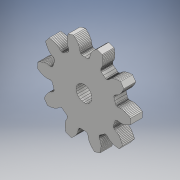
# Autodesk Inventor part: Engranajes PEQUENO final 2017
Saved by Autodesk Inventor 2017 (Build 210142000, 142)
## iProperties
Created: 2017-09-24
Part Number: Engranajes PEQUENO final 2017
Material: Generic
Document SubType Name: Modeling
Designer: ANDRES
Density: 1 g/cm^3
Appearance: Default
Author: ANDRES
## iProperties of the stored document Engranajes PEQUENO final 2017_3DPrint.ipt
Created: 2017-09-24
Part Number: Engranajes PEQUENO final 2017_3DPrint
Material: Generic
Document SubType Name: Modeling
Designer: ANDRES
Density: 1 g/cm^3
Appearance: Default
Author: ANDRES
Autodesk Inventor part; units mm, degrees
ref_plane "YZ Plane" through (0, 0, 0) normal (1, 0, 0) x (0, 1, 0)
ref_plane "XZ Plane" through (0, 0, 0) normal (0, 1, 0) x (-1, 0, 0)
ref_plane "XY Plane" through (0, 0, 0) normal (0, 0, 1) x (1, 0, 0)
sketch "Sketch1" plane through (0, 0, 0) normal (0, 1, 0) x (-1, 0, 0)
  line L0 (3.2222, 8) -> (3.1344, 8.1445)
  line L1 (3.1344, 8.1445) -> (3.0716, 8.1935)
  line L2 (3.0716, 8.1935) -> (3.0129, 8.2255)
  line L3 (3.0129, 8.2255) -> (2.9568, 8.2486)
  line L4 (2.9568, 8.2486) -> (2.902, 8.2657)
  line L5 (2.902, 8.2657) -> (2.8484, 8.2779)
  line L6 (2.8484, 8.2779) -> (2.7432, 8.2923)
  line L7 (2.7432, 8.2923) -> (2.6406, 8.2961)
  line L8 (2.6406, 8.2961) -> (2.5395, 8.2918)
  line L9 (2.5395, 8.2918) -> (2.3414, 8.2639)
  line L10 (2.3414, 8.2639) -> (2.1473, 8.2146)
  line L11 (2.1473, 8.2146) -> (1.9461, 8.2027)
  line L12 (1.9461, 8.2027) -> (1.7394, 8.2197)
  line L13 (1.7394, 8.2197) -> (1.5296, 8.2547)
  line L14 (1.5296, 8.2547) -> (1.318, 8.3058)
  line L15 (1.318, 8.3058) -> (1.1049, 8.3713)
  line L16 (1.1049, 8.3713) -> (0.8908, 8.4503)
  line L17 (0.8908, 8.4503) -> (0.6767, 8.5423)
  line L18 (0.6767, 8.5423) -> (0.4623, 8.6469)
  line L19 (0.4623, 8.6469) -> (0.2484, 8.7638)
  line L20 (0.2484, 8.7638) -> (0.0358, 8.8928)
  line L21 (0.0358, 8.8928) -> (0.0061, 10.0714)
  line L22 (0.0061, 10.0714) -> (0.2121, 10.2108)
  line L23 (0.2121, 10.2108) -> (0.4199, 10.3383)
  line L24 (0.4199, 10.3383) -> (0.6284, 10.4534)
  line L25 (0.6284, 10.4534) -> (0.8379, 10.5562)
  line L26 (0.8379, 10.5562) -> (1.0478, 10.6459)
  line L27 (1.0478, 10.6459) -> (1.2573, 10.7218)
  line L28 (1.2573, 10.7218) -> (1.4661, 10.7836)
  line L29 (1.4661, 10.7836) -> (1.6739, 10.8293)
  line L30 (1.6739, 10.8293) -> (1.8793, 10.8565)
  line L31 (1.8793, 10.8565) -> (2.081, 10.8547)
  line L32 (2.081, 10.8547) -> (2.2771, 10.8153)
  line L33 (2.2771, 10.8153) -> (2.4765, 10.7973)
  line L34 (2.4765, 10.7973) -> (2.5776, 10.798)
  line L35 (2.5776, 10.798) -> (2.68, 10.8069)
  line L36 (2.68, 10.8069) -> (2.7843, 10.8268)
  line L37 (2.7843, 10.8268) -> (2.8372, 10.8417)
  line L38 (2.8372, 10.8417) -> (2.891, 10.8613)
  line L39 (2.891, 10.8613) -> (2.9461, 10.8872)
  line L40 (2.9461, 10.8872) -> (3.003, 10.9223)
  line L41 (3.003, 10.9223) -> (3.0632, 10.9743)
  line L42 (3.0632, 10.9743) -> (3.1438, 11.1229)
  line L43 (3.1438, 11.1229) -> (3.2763, 11.6439)
  line L44 (3.2763, 11.6439) -> (3.4498, 12.1524)
  line L45 (3.4498, 12.1524) -> (3.4635, 12.321)
  line L46 (3.4635, 12.321) -> (3.4417, 12.3975)
  line L47 (3.4417, 12.3975) -> (3.4133, 12.4579)
  line L48 (3.4133, 12.4579) -> (3.3812, 12.5098)
  line L49 (3.3812, 12.5098) -> (3.347, 12.5555)
  line L50 (3.347, 12.5555) -> (3.3106, 12.5971)
  line L51 (3.3106, 12.5971) -> (3.2342, 12.6705)
  line L52 (3.2342, 12.6705) -> (3.1534, 12.734)
  line L53 (3.1534, 12.734) -> (3.0691, 12.7899)
  line L54 (3.0691, 12.7899) -> (2.8923, 12.8836)
  line L55 (2.8923, 12.8836) -> (2.7064, 12.9578)
  line L56 (2.7064, 12.9578) -> (2.5364, 13.0665)
  line L57 (2.5364, 13.0665) -> (2.3792, 13.2017)
  line L58 (2.3792, 13.2017) -> (2.2304, 13.3535)
  line L59 (2.2304, 13.3535) -> (2.0892, 13.5191)
  line L60 (2.0892, 13.5191) -> (1.955, 13.6975)
  line L61 (1.955, 13.6975) -> (1.8283, 13.8872)
  line L62 (1.8283, 13.8872) -> (1.7092, 14.0876)
  line L63 (1.7092, 14.0876) -> (1.5972, 14.2982)
  line L64 (1.5972, 14.2982) -> (1.493, 14.5184)
  line L65 (1.493, 14.5184) -> (1.3967, 14.7477)
  line L66 (1.3967, 14.7477) -> (2.0655, 15.7185)
  line L67 (2.0655, 15.7185) -> (2.3142, 15.7104)
  line L68 (2.3142, 15.7104) -> (2.557, 15.6914)
  line L69 (2.557, 15.6914) -> (2.7935, 15.6619)
  line L70 (2.7935, 15.6619) -> (3.0234, 15.622)
  line L71 (3.0234, 15.622) -> (3.2459, 15.5712)
  line L72 (3.2459, 15.5712) -> (3.46, 15.5095)
  line L73 (3.46, 15.5095) -> (3.6652, 15.4366)
  line L74 (3.6652, 15.4366) -> (3.86, 15.3515)
  line L75 (3.86, 15.3515) -> (4.0424, 15.2527)
  line L76 (4.0424, 15.2527) -> (4.2044, 15.1328)
  line L77 (4.2044, 15.1328) -> (4.3401, 14.9855)
  line L78 (4.3401, 14.9855) -> (4.4907, 14.8539)
  line L79 (4.4907, 14.8539) -> (4.573, 14.7949)
  line L80 (4.573, 14.7949) -> (4.6611, 14.7421)
  line L81 (4.6611, 14.7421) -> (4.7569, 14.6966)
  line L82 (4.7569, 14.6966) -> (4.8087, 14.6776)
  line L83 (4.8087, 14.6776) -> (4.8638, 14.6618)
  line L84 (4.8638, 14.6618) -> (4.9235, 14.6504)
  line L85 (4.9235, 14.6504) -> (4.99, 14.6456)
  line L86 (4.99, 14.6456) -> (5.0695, 14.6522)
  line L87 (5.0695, 14.6522) -> (5.2219, 14.725)
  line L88 (5.2219, 14.725) -> (5.6355, 15.0684)
  line L89 (5.6355, 15.0684) -> (6.0747, 15.3778)
  line L90 (6.0747, 15.3778) -> (6.1849, 15.506)
  line L91 (6.1849, 15.506) -> (6.2121, 15.581)
  line L92 (6.2121, 15.581) -> (6.2245, 15.6467)
  line L93 (6.2245, 15.6467) -> (6.2291, 15.7072)
  line L94 (6.2291, 15.7072) -> (6.2283, 15.7646)
  line L95 (6.2283, 15.7646) -> (6.2234, 15.8195)
  line L96 (6.2234, 15.8195) -> (6.2046, 15.9239)
  line L97 (6.2046, 15.9239) -> (6.1767, 16.0227)
  line L98 (6.1767, 16.0227) -> (6.1411, 16.1174)
  line L99 (6.1411, 16.1174) -> (6.0532, 16.2972)
  line L100 (6.0532, 16.2972) -> (5.9464, 16.4663)
  line L101 (5.9464, 16.4663) -> (5.873, 16.6543)
  line L102 (5.873, 16.6543) -> (5.8249, 16.856)
  line L103 (5.8249, 16.856) -> (5.7937, 17.0663)
  line L104 (5.7937, 17.0663) -> (5.7768, 17.2834)
  line L105 (5.7768, 17.2834) -> (5.773, 17.5064)
  line L106 (5.773, 17.5064) -> (5.7821, 17.7343)
  line L107 (5.7821, 17.7343) -> (5.8034, 17.9664)
  line L108 (5.8034, 17.9664) -> (5.8366, 18.2027)
  line L109 (5.8366, 18.2027) -> (5.8815, 18.4419)
  line L110 (5.8815, 18.4419) -> (5.9383, 18.6843)
  line L111 (5.9383, 18.6843) -> (7.05, 19.0769)
  line L112 (7.05, 19.0769) -> (7.2464, 18.9241)
  line L113 (7.2464, 18.9241) -> (7.4318, 18.7661)
  line L114 (7.4318, 18.7661) -> (7.6059, 18.6031)
  line L115 (7.6059, 18.6031) -> (7.7685, 18.4358)
  line L116 (7.7685, 18.4358) -> (7.9184, 18.2641)
  line L117 (7.9184, 18.2641) -> (8.0556, 18.0883)
  line L118 (8.0556, 18.0883) -> (8.1788, 17.9088)
  line L119 (8.1788, 17.9088) -> (8.2865, 17.7254)
  line L120 (8.2865, 17.7254) -> (8.376, 17.5383)
  line L121 (8.376, 17.5383) -> (8.4367, 17.346)
  line L122 (8.4367, 17.346) -> (8.4599, 17.1471)
  line L123 (8.4599, 17.1471) -> (8.5044, 16.952)
  line L124 (8.5044, 16.952) -> (8.5364, 16.856)
  line L125 (8.5364, 16.856) -> (8.5765, 16.7616)
  line L126 (8.5765, 16.7616) -> (8.6274, 16.6686)
  line L127 (8.6274, 16.6686) -> (8.6581, 16.6226)
  line L128 (8.6581, 16.6226) -> (8.6934, 16.5777)
  line L129 (8.6934, 16.5777) -> (8.7351, 16.5333)
  line L130 (8.7351, 16.5333) -> (8.7859, 16.4901)
  line L131 (8.7859, 16.4901) -> (8.8542, 16.4489)
  line L132 (8.8542, 16.4489) -> (9.0204, 16.4183)
  line L133 (9.0204, 16.4183) -> (9.5568, 16.4532)
  line L134 (9.5568, 16.4532) -> (10.094, 16.4454)
  line L135 (10.094, 16.4454) -> (10.2586, 16.4845)
  line L136 (10.2586, 16.4845) -> (10.3246, 16.529)
  line L137 (10.3246, 16.529) -> (10.3734, 16.5747)
  line L138 (10.3734, 16.5747) -> (10.4125, 16.6212)
  line L139 (10.4125, 16.6212) -> (10.4455, 16.6679)
  line L140 (10.4455, 16.6679) -> (10.474, 16.7152)
  line L141 (10.474, 16.7152) -> (10.5199, 16.8107)
  line L142 (10.5199, 16.8107) -> (10.5555, 16.9072)
  line L143 (10.5555, 16.9072) -> (10.5826, 17.0048)
  line L144 (10.5826, 17.0048) -> (10.6171, 17.2019)
  line L145 (10.6171, 17.2019) -> (10.6301, 17.4015)
  line L146 (10.6301, 17.4015) -> (10.6811, 17.5966)
  line L147 (10.6811, 17.5966) -> (10.7611, 17.7881)
  line L148 (10.7611, 17.7881) -> (10.8593, 17.9766)
  line L149 (10.8593, 17.9766) -> (10.9731, 18.1621)
  line L150 (10.9731, 18.1621) -> (11.1011, 18.3447)
  line L151 (11.1011, 18.3447) -> (11.2425, 18.5238)
  line L152 (11.2425, 18.5238) -> (11.3962, 18.6993)
  line L153 (11.3962, 18.6993) -> (11.5617, 18.8708)
  line L154 (11.5617, 18.8708) -> (11.7391, 19.0379)
  line L155 (11.7391, 19.0379) -> (11.9273, 19.2002)
  line L156 (11.9273, 19.2002) -> (13.0576, 18.8643)
  line L157 (13.0576, 18.8643) -> (13.1264, 18.6251)
  line L158 (13.1264, 18.6251) -> (13.1835, 18.3883)
  line L159 (13.1835, 18.3883) -> (13.2284, 18.1542)
  line L160 (13.2284, 18.1542) -> (13.2614, 17.9233)
  line L161 (13.2614, 17.9233) -> (13.2821, 17.6962)
  line L162 (13.2821, 17.6962) -> (13.2895, 17.4732)
  line L163 (13.2895, 17.4732) -> (13.2837, 17.2555)
  line L164 (13.2837, 17.2555) -> (13.2629, 17.0439)
  line L165 (13.2629, 17.0439) -> (13.2253, 16.8402)
  line L166 (13.2253, 16.8402) -> (13.1613, 16.6487)
  line L167 (13.1613, 16.6487) -> (13.0633, 16.4744)
  line L168 (13.0633, 16.4744) -> (12.9846, 16.2905)
  line L169 (12.9846, 16.2905) -> (12.9541, 16.194)
  line L170 (12.9541, 16.194) -> (12.931, 16.0939)
  line L171 (12.931, 16.0939) -> (12.9176, 15.9887)
  line L172 (12.9176, 15.9887) -> (12.9156, 15.9336)
  line L173 (12.9156, 15.9336) -> (12.9176, 15.8762)
  line L174 (12.9176, 15.8762) -> (12.9252, 15.816)
  line L175 (12.9252, 15.816) -> (12.941, 15.751)
  line L176 (12.941, 15.751) -> (12.972, 15.6776)
  line L177 (12.972, 15.6776) -> (13.0884, 15.5549)
  line L178 (13.0884, 15.5549) -> (13.5428, 15.2682)
  line L179 (13.5428, 15.2682) -> (13.9729, 14.946)
  line L180 (13.9729, 14.946) -> (14.1288, 14.881)
  line L181 (14.1288, 14.881) -> (14.2086, 14.8782)
  line L182 (14.2086, 14.8782) -> (14.2749, 14.8866)
  line L183 (14.2749, 14.8866) -> (14.3341, 14.9011)
  line L184 (14.3341, 14.9011) -> (14.3882, 14.9194)
  line L185 (14.3882, 14.9194) -> (14.439, 14.941)
  line L186 (14.439, 14.941) -> (14.5322, 14.9913)
  line L187 (14.5322, 14.9913) -> (14.6178, 15.0485)
  line L188 (14.6178, 15.0485) -> (14.6968, 15.1115)
  line L189 (14.6968, 15.1115) -> (14.8407, 15.2507)
  line L190 (14.8407, 15.2507) -> (14.9687, 15.4044)
  line L191 (14.9687, 15.4044) -> (15.1244, 15.5324)
  line L192 (15.1244, 15.5324) -> (15.3017, 15.6401)
  line L193 (15.3017, 15.6401) -> (15.4919, 15.7349)
  line L194 (15.4919, 15.7349) -> (15.6931, 15.8182)
  line L195 (15.6931, 15.8182) -> (15.9042, 15.8907)
  line L196 (15.9042, 15.8907) -> (16.1236, 15.9524)
  line L197 (16.1236, 15.9524) -> (16.3512, 16.004)
  line L198 (16.3512, 16.004) -> (16.5859, 16.0455)
  line L199 (16.5859, 16.0455) -> (16.8277, 16.0765)
  line L200 (16.8277, 16.0765) -> (17.0756, 16.0974)
  line L201 (17.0756, 16.0974) -> (17.7923, 15.1612)
  line L202 (17.7923, 15.1612) -> (17.7077, 14.9273)
  line L203 (17.7077, 14.9273) -> (17.6148, 14.7022)
  line L204 (17.6148, 14.7022) -> (17.5135, 14.4863)
  line L205 (17.5135, 14.4863) -> (17.4045, 14.28)
  line L206 (17.4045, 14.28) -> (17.2875, 14.0842)
  line L207 (17.2875, 14.0842) -> (17.1628, 13.8995)
  line L208 (17.1628, 13.8995) -> (17.03, 13.727)
  line L209 (17.03, 13.727) -> (16.889, 13.5677)
  line L210 (16.889, 13.5677) -> (16.7387, 13.425)
  line L211 (16.7387, 13.425) -> (16.5744, 13.3078)
  line L212 (16.5744, 13.3078) -> (16.3925, 13.2242)
  line L213 (16.3925, 13.2242) -> (16.2208, 13.1219)
  line L214 (16.2208, 13.1219) -> (16.1393, 13.0616)
  line L215 (16.1393, 13.0616) -> (16.0619, 12.9941)
  line L216 (16.0619, 12.9941) -> (15.9892, 12.9171)
  line L217 (15.9892, 12.9171) -> (15.9552, 12.8737)
  line L218 (15.9552, 12.8737) -> (15.9232, 12.8261)
  line L219 (15.9232, 12.8261) -> (15.8937, 12.7728)
  line L220 (15.8937, 12.7728) -> (15.8684, 12.7111)
  line L221 (15.8684, 12.7111) -> (15.8503, 12.6336)
  line L222 (15.8503, 12.6336) -> (15.8725, 12.466)
  line L223 (15.8725, 12.466) -> (16.0714, 11.9666)
  line L224 (16.0714, 11.9666) -> (16.2299, 11.4533)
  line L225 (16.2299, 11.4533) -> (16.3181, 11.3088)
  line L226 (16.3181, 11.3088) -> (16.3808, 11.2598)
  line L227 (16.3808, 11.2598) -> (16.4395, 11.2275)
  line L228 (16.4395, 11.2275) -> (16.4956, 11.2046)
  line L229 (16.4956, 11.2046) -> (16.5505, 11.1876)
  line L230 (16.5505, 11.1876) -> (16.6041, 11.1752)
  line L231 (16.6041, 11.1752) -> (16.709, 11.161)
  line L232 (16.709, 11.161) -> (16.8118, 11.1571)
  line L233 (16.8118, 11.1571) -> (16.9129, 11.1615)
  line L234 (16.9129, 11.1615) -> (17.1111, 11.1894)
  line L235 (17.1111, 11.1894) -> (17.3049, 11.2387)
  line L236 (17.3049, 11.2387) -> (17.5063, 11.2504)
  line L237 (17.5063, 11.2504) -> (17.713, 11.2336)
  line L238 (17.713, 11.2336) -> (17.9226, 11.1983)
  line L239 (17.9226, 11.1983) -> (18.1344, 11.1472)
  line L240 (18.1344, 11.1472) -> (18.3475, 11.082)
  line L241 (18.3475, 11.082) -> (18.5614, 11.003)
  line L242 (18.5614, 11.003) -> (18.7758, 10.9108)
  line L243 (18.7758, 10.9108) -> (18.9902, 10.8064)
  line L244 (18.9902, 10.8064) -> (19.2038, 10.6893)
  line L245 (19.2038, 10.6893) -> (19.4166, 10.5605)
  line L246 (19.4166, 10.5605) -> (19.4463, 9.3819)
  line L247 (19.4463, 9.3819) -> (19.2401, 9.243)
  line L248 (19.2401, 9.243) -> (19.0326, 9.1155)
  line L249 (19.0326, 9.1155) -> (18.8238, 9.0001)
  line L250 (18.8238, 9.0001) -> (18.6145, 8.8975)
  line L251 (18.6145, 8.8975) -> (18.4047, 8.8079)
  line L252 (18.4047, 8.8079) -> (18.1951, 8.7319)
  line L253 (18.1951, 8.7319) -> (17.9864, 8.6702)
  line L254 (17.9864, 8.6702) -> (17.7786, 8.6245)
  line L255 (17.7786, 8.6245) -> (17.5731, 8.5973)
  line L256 (17.5731, 8.5973) -> (17.3714, 8.5991)
  line L257 (17.3714, 8.5991) -> (17.1751, 8.6384)
  line L258 (17.1751, 8.6384) -> (16.9759, 8.6565)
  line L259 (16.9759, 8.6565) -> (16.8749, 8.6557)
  line L260 (16.8749, 8.6557) -> (16.7722, 8.6466)
  line L261 (16.7722, 8.6466) -> (16.6681, 8.627)
  line L262 (16.6681, 8.627) -> (16.6153, 8.612)
  line L263 (16.6153, 8.612) -> (16.5614, 8.5925)
  line L264 (16.5614, 8.5925) -> (16.5063, 8.5666)
  line L265 (16.5063, 8.5666) -> (16.4494, 8.5315)
  line L266 (16.4494, 8.5315) -> (16.3892, 8.4792)
  line L267 (16.3892, 8.4792) -> (16.3084, 8.3306)
  line L268 (16.3084, 8.3306) -> (16.1761, 7.8099)
  line L269 (16.1761, 7.8099) -> (16.0024, 7.3014)
  line L270 (16.0024, 7.3014) -> (15.9886, 7.1327)
  line L271 (15.9886, 7.1327) -> (16.0107, 7.0563)
  line L272 (16.0107, 7.0563) -> (16.0392, 6.9958)
  line L273 (16.0392, 6.9958) -> (16.0712, 6.944)
  line L274 (16.0712, 6.944) -> (16.1055, 6.898)
  line L275 (16.1055, 6.898) -> (16.1418, 6.8566)
  line L276 (16.1418, 6.8566) -> (16.2183, 6.7832)
  line L277 (16.2183, 6.7832) -> (16.299, 6.7197)
  line L278 (16.299, 6.7197) -> (16.3834, 6.6638)
  line L279 (16.3834, 6.6638) -> (16.5601, 6.5701)
  line L280 (16.5601, 6.5701) -> (16.7461, 6.4957)
  line L281 (16.7461, 6.4957) -> (16.9157, 6.387)
  line L282 (16.9157, 6.387) -> (17.0732, 6.2519)
  line L283 (17.0732, 6.2519) -> (17.2221, 6.1002)
  line L284 (17.2221, 6.1002) -> (17.3633, 5.9346)
  line L285 (17.3633, 5.9346) -> (17.4974, 5.7563)
  line L286 (17.4974, 5.7563) -> (17.6239, 5.5666)
  line L287 (17.6239, 5.5666) -> (17.7433, 5.3662)
  line L288 (17.7433, 5.3662) -> (17.855, 5.1556)
  line L289 (17.855, 5.1556) -> (17.9594, 4.9354)
  line L290 (17.9594, 4.9354) -> (18.0557, 4.706)
  line L291 (18.0557, 4.706) -> (17.3869, 3.735)
  line L292 (17.3869, 3.735) -> (17.1383, 3.7434)
  line L293 (17.1383, 3.7434) -> (16.8954, 3.7624)
  line L294 (16.8954, 3.7624) -> (16.6587, 3.7919)
  line L295 (16.6587, 3.7919) -> (16.4291, 3.8317)
  line L296 (16.4291, 3.8317) -> (16.2066, 3.8825)
  line L297 (16.2066, 3.8825) -> (15.9925, 3.9443)
  line L298 (15.9925, 3.9443) -> (15.7872, 4.0172)
  line L299 (15.7872, 4.0172) -> (15.5924, 4.1023)
  line L300 (15.5924, 4.1023) -> (15.41, 4.2011)
  line L301 (15.41, 4.2011) -> (15.248, 4.321)
  line L302 (15.248, 4.321) -> (15.1124, 4.4681)
  line L303 (15.1124, 4.4681) -> (14.9618, 4.5999)
  line L304 (14.9618, 4.5999) -> (14.8795, 4.6588)
  line L305 (14.8795, 4.6588) -> (14.7913, 4.7117)
  line L306 (14.7913, 4.7117) -> (14.6956, 4.7571)
  line L307 (14.6956, 4.7571) -> (14.6438, 4.7759)
  line L308 (14.6438, 4.7759) -> (14.5886, 4.7917)
  line L309 (14.5886, 4.7917) -> (14.529, 4.8031)
  line L310 (14.529, 4.8031) -> (14.4624, 4.8082)
  line L311 (14.4624, 4.8082) -> (14.3829, 4.8016)
  line L312 (14.3829, 4.8016) -> (14.2303, 4.7287)
  line L313 (14.2303, 4.7287) -> (13.8171, 4.3852)
  line L314 (13.8171, 4.3852) -> (13.3777, 4.0754)
  line L315 (13.3777, 4.0754) -> (13.2678, 3.9471)
  line L316 (13.2678, 3.9471) -> (13.2406, 3.8722)
  line L317 (13.2406, 3.8722) -> (13.2279, 3.8067)
  line L318 (13.2279, 3.8067) -> (13.2234, 3.746)
  line L319 (13.2234, 3.746) -> (13.2244, 3.6888)
  line L320 (13.2244, 3.6888) -> (13.2292, 3.6339)
  line L321 (13.2292, 3.6339) -> (13.2481, 3.5296)
  line L322 (13.2481, 3.5296) -> (13.276, 3.4308)
  line L323 (13.276, 3.4308) -> (13.3113, 3.3358)
  line L324 (13.3113, 3.3358) -> (13.3995, 3.1562)
  line L325 (13.3995, 3.1562) -> (13.5062, 2.9868)
  line L326 (13.5062, 2.9868) -> (13.5796, 2.7991)
  line L327 (13.5796, 2.7991) -> (13.6274, 2.5972)
  line L328 (13.6274, 2.5972) -> (13.6587, 2.3871)
  line L329 (13.6587, 2.3871) -> (13.6757, 2.1699)
  line L330 (13.6757, 2.1699) -> (13.6793, 1.9469)
  line L331 (13.6793, 1.9469) -> (13.6704, 1.7191)
  line L332 (13.6704, 1.7191) -> (13.6491, 1.4867)
  line L333 (13.6491, 1.4867) -> (13.6159, 1.2507)
  line L334 (13.6159, 1.2507) -> (13.5707, 1.0112)
  line L335 (13.5707, 1.0112) -> (13.5142, 0.7691)
  line L336 (13.5142, 0.7691) -> (12.4025, 0.3764)
  line L337 (12.4025, 0.3764) -> (12.2061, 0.5293)
  line L338 (12.2061, 0.5293) -> (12.0207, 0.6872)
  line L339 (12.0207, 0.6872) -> (11.8464, 0.85)
  line L340 (11.8464, 0.85) -> (11.684, 1.0176)
  line L341 (11.684, 1.0176) -> (11.5339, 1.1893)
  line L342 (11.5339, 1.1893) -> (11.3969, 1.365)
  line L343 (11.3969, 1.365) -> (11.2737, 1.5446)
  line L344 (11.2737, 1.5446) -> (11.166, 1.728)
  line L345 (11.166, 1.728) -> (11.0765, 1.9151)
  line L346 (11.0765, 1.9151) -> (11.0158, 2.1074)
  line L347 (11.0158, 2.1074) -> (10.9926, 2.306)
  line L348 (10.9926, 2.306) -> (10.9481, 2.5013)
  line L349 (10.9481, 2.5013) -> (10.9161, 2.5971)
  line L350 (10.9161, 2.5971) -> (10.876, 2.6918)
  line L351 (10.876, 2.6918) -> (10.8251, 2.7848)
  line L352 (10.8251, 2.7848) -> (10.7944, 2.8305)
  line L353 (10.7944, 2.8305) -> (10.7591, 2.8757)
  line L354 (10.7591, 2.8757) -> (10.7174, 2.9199)
  line L355 (10.7174, 2.9199) -> (10.6664, 2.9633)
  line L356 (10.6664, 2.9633) -> (10.5983, 3.0045)
  line L357 (10.5983, 3.0045) -> (10.4319, 3.0352)
  line L358 (10.4319, 3.0352) -> (9.8957, 3.0002)
  line L359 (9.8957, 3.0002) -> (9.3585, 3.0083)
  line L360 (9.3585, 3.0083) -> (9.1939, 2.9692)
  line L361 (9.1939, 2.9692) -> (9.1279, 2.9245)
  line L362 (9.1279, 2.9245) -> (9.0791, 2.8787)
  line L363 (9.0791, 2.8787) -> (9.0398, 2.8325)
  line L364 (9.0398, 2.8325) -> (9.0068, 2.7855)
  line L365 (9.0068, 2.7855) -> (8.9786, 2.7382)
  line L366 (8.9786, 2.7382) -> (8.9324, 2.643)
  line L367 (8.9324, 2.643) -> (8.8971, 2.5465)
  line L368 (8.8971, 2.5465) -> (8.8699, 2.4489)
  line L369 (8.8699, 2.4489) -> (8.8354, 2.2518)
  line L370 (8.8354, 2.2518) -> (8.8222, 2.0522)
  line L371 (8.8222, 2.0522) -> (8.7715, 1.8571)
  line L372 (8.7715, 1.8571) -> (8.6915, 1.6656)
  line L373 (8.6915, 1.6656) -> (8.5932, 1.4771)
  line L374 (8.5932, 1.4771) -> (8.4795, 1.2914)
  line L375 (8.4795, 1.2914) -> (8.3512, 1.109)
  line L376 (8.3512, 1.109) -> (8.21, 0.9299)
  line L377 (8.21, 0.9299) -> (8.0564, 0.7544)
  line L378 (8.0564, 0.7544) -> (7.8905, 0.5829)
  line L379 (7.8905, 0.5829) -> (7.7135, 0.4157)
  line L380 (7.7135, 0.4157) -> (7.5251, 0.2531)
  line L381 (7.5251, 0.2531) -> (6.395, 0.589)
  line L382 (6.395, 0.589) -> (6.3261, 0.828)
  line L383 (6.3261, 0.828) -> (6.2689, 1.065)
  line L384 (6.2689, 1.065) -> (6.2237, 1.2989)
  line L385 (6.2237, 1.2989) -> (6.1909, 1.53)
  line L386 (6.1909, 1.53) -> (6.1703, 1.7571)
  line L387 (6.1703, 1.7571) -> (6.1626, 1.9798)
  line L388 (6.1626, 1.9798) -> (6.1687, 2.1975)
  line L389 (6.1687, 2.1975) -> (6.1892, 2.4091)
  line L390 (6.1892, 2.4091) -> (6.227, 2.6131)
  line L391 (6.227, 2.6131) -> (6.2907, 2.8044)
  line L392 (6.2907, 2.8044) -> (6.3888, 2.9789)
  line L393 (6.3888, 2.9789) -> (6.4677, 3.1628)
  line L394 (6.4677, 3.1628) -> (6.4982, 3.2593)
  line L395 (6.4982, 3.2593) -> (6.5213, 3.3594)
  line L396 (6.5213, 3.3594) -> (6.5347, 3.4645)
  line L397 (6.5347, 3.4645) -> (6.5368, 3.5197)
  line L398 (6.5368, 3.5197) -> (6.5347, 3.5768)
  line L399 (6.5347, 3.5768) -> (6.5271, 3.6373)
  line L400 (6.5271, 3.6373) -> (6.5113, 3.702)
  line L401 (6.5113, 3.702) -> (6.4803, 3.7757)
  line L402 (6.4803, 3.7757) -> (6.364, 3.8981)
  line L403 (6.364, 3.8981) -> (5.9095, 4.185)
  line L404 (5.9095, 4.185) -> (5.4794, 4.5073)
  line L405 (5.4794, 4.5073) -> (5.3232, 4.5723)
  line L406 (5.3232, 4.5723) -> (5.2437, 4.5751)
  line L407 (5.2437, 4.5751) -> (5.1774, 4.5667)
  line L408 (5.1774, 4.5667) -> (5.1182, 4.5522)
  line L409 (5.1182, 4.5522) -> (5.0641, 4.5336)
  line L410 (5.0641, 4.5336) -> (5.0134, 4.512)
  line L411 (5.0134, 4.512) -> (4.9199, 4.462)
  line L412 (4.9199, 4.462) -> (4.8346, 4.4048)
  line L413 (4.8346, 4.4048) -> (4.7553, 4.3418)
  line L414 (4.7553, 4.3418) -> (4.6116, 4.2026)
  line L415 (4.6116, 4.2026) -> (4.4836, 4.0489)
  line L416 (4.4836, 4.0489) -> (4.3276, 3.9209)
  line L417 (4.3276, 3.9209) -> (4.1506, 3.8129)
  line L418 (4.1506, 3.8129) -> (3.9604, 3.7181)
  line L419 (3.9604, 3.7181) -> (3.759, 3.635)
  line L420 (3.759, 3.635) -> (3.5482, 3.5626)
  line L421 (3.5482, 3.5626) -> (3.3287, 3.5008)
  line L422 (3.3287, 3.5008) -> (3.1012, 3.4492)
  line L423 (3.1012, 3.4492) -> (2.8662, 3.4078)
  line L424 (2.8662, 3.4078) -> (2.6247, 3.3768)
  line L425 (2.6247, 3.3768) -> (2.3768, 3.3559)
  line L426 (2.3768, 3.3559) -> (1.6598, 4.2918)
  line L427 (1.6598, 4.2918) -> (1.7446, 4.5257)
  line L428 (1.7446, 4.5257) -> (1.8376, 4.751)
  line L429 (1.8376, 4.751) -> (1.9386, 4.967)
  line L430 (1.9386, 4.967) -> (2.0478, 5.1732)
  line L431 (2.0478, 5.1732) -> (2.1646, 5.3688)
  line L432 (2.1646, 5.3688) -> (2.2895, 5.5538)
  line L433 (2.2895, 5.5538) -> (2.4224, 5.7262)
  line L434 (2.4224, 5.7262) -> (2.5633, 5.8853)
  line L435 (2.5633, 5.8853) -> (2.7136, 6.0283)
  line L436 (2.7136, 6.0283) -> (2.8777, 6.1454)
  line L437 (2.8777, 6.1454) -> (3.0596, 6.229)
  line L438 (3.0596, 6.229) -> (3.2315, 6.3314)
  line L439 (3.2315, 6.3314) -> (3.3128, 6.3916)
  line L440 (3.3128, 6.3916) -> (3.3905, 6.4589)
  line L441 (3.3905, 6.4589) -> (3.4631, 6.5362)
  line L442 (3.4631, 6.5362) -> (3.4971, 6.5793)
  line L443 (3.4971, 6.5793) -> (3.5291, 6.6271)
  line L444 (3.5291, 6.6271) -> (3.5583, 6.6802)
  line L445 (3.5583, 6.6802) -> (3.5837, 6.7422)
  line L446 (3.5837, 6.7422) -> (3.602, 6.8196)
  line L447 (3.602, 6.8196) -> (3.5799, 6.9873)
  line L448 (3.5799, 6.9873) -> (3.3807, 7.4867)
  line L449 (3.3807, 7.4867) -> (3.2222, 8)
  line L450 (11.377, 9.726) -> (11.3208, 10.1534)
  line L451 (11.3208, 10.1534) -> (11.156, 10.5514)
  line L452 (11.156, 10.5514) -> (10.8936, 10.8936)
  line L453 (10.8936, 10.8936) -> (10.5514, 11.1559)
  line L454 (10.5514, 11.1559) -> (10.1534, 11.3208)
  line L455 (10.1534, 11.3208) -> (9.7259, 11.3769)
  line L456 (9.7259, 11.3769) -> (9.2987, 11.3208)
  line L457 (9.2987, 11.3208) -> (8.9004, 11.1559)
  line L458 (8.9004, 11.1559) -> (8.5585, 10.8936)
  line L459 (8.5585, 10.8936) -> (8.2961, 10.5514)
  line L460 (8.2961, 10.5514) -> (8.1313, 10.1534)
  line L461 (8.1313, 10.1534) -> (8.0749, 9.7259)
  line L462 (8.0749, 9.7259) -> (8.1313, 9.2987)
  line L463 (8.1313, 9.2987) -> (8.2961, 8.9004)
  line L464 (8.2961, 8.9004) -> (8.5585, 8.5585)
  line L465 (8.5585, 8.5585) -> (8.9004, 8.2961)
  line L466 (8.9004, 8.2961) -> (9.2987, 8.1313)
  line L467 (9.2987, 8.1313) -> (9.7263, 8.0749)
  line L468 (9.7263, 8.0749) -> (10.1536, 8.1313)
  line L469 (10.1536, 8.1313) -> (10.5516, 8.2962)
  line L470 (10.5516, 8.2962) -> (10.8937, 8.5586)
  line L471 (10.8937, 8.5586) -> (11.1561, 8.9005)
  line L472 (11.1561, 8.9005) -> (11.3209, 9.2987)
  line L473 (11.3209, 9.2987) -> (11.377, 9.726)
  point P0 (0, 0)
  constraints: 948 end point, 80 parallel, 23 perpendicular
extrude "Extrusion1" add sketch "Sketch1" along normal blind 2.5
body "Solid1"
